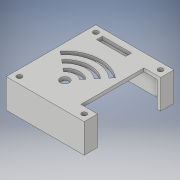
# Autodesk Inventor part: Box1_Top
Saved by Autodesk Inventor 2017 (Build 210142000, 142)
## iProperties
Created: 2017-11-12
Part Number: Box1_Top
Material: Generic
Document SubType Name: Modeling
Designer: Arthur Bondar
Density: 1 g/cm^3
Appearance: Default
Author: Arthur Bondar
Autodesk Inventor part; units mm, degrees
ref_plane "YZ Plane" through (0, 0, 0) normal (1, 0, 0) x (0, 1, 0)
ref_plane "XZ Plane" through (0, 0, 0) normal (0, 1, 0) x (-1, 0, 0)
ref_plane "XY Plane" through (0, 0, 0) normal (0, 0, 1) x (1, 0, 0)
sketch "Sketch1" plane through (0, 0, 0) normal (0, 1, 0) x (-1, 0, 0)
  line L0 (23.5, 27) -> (-23.5, 27)
  line L1 (-23.5, -27) -> (23.5, -27)
  line L2 (23.5, -27) -> (23.5, 27)
  line L3 (21.5, 25) -> (-21.5, 25)
  line L4 (-21.5, -25) -> (21.5, -25)
  line L5 (21.5, -25) -> (21.5, 25)
  line L6 (-21.5, -25) -> (-21.5, -19)
  line L7 (-21.5, -19) -> (-23.5, -19)
  line L8 (-21.5, 25) -> (-21.5, 19)
  line L9 (-21.5, 19) -> (-23.5, 19)
  line L10 (-23.5, 27) -> (-23.5, 19)
  line L11 (-23.5, -19) -> (-23.5, -27)
  line L12 (-21.5, 25) -> (-21.5, 19)
  line L13 (-21.5, -19) -> (-21.5, -25)
  dimension "d2" = 47
  dimension "d3" = 54
  dimension "d4" = 43
  dimension "d5" = 50
  dimension "d6" = 6
  dimension "d7" = 6
  constraints: 28 end point, 8 perpendicular, 6 parallel, 2 horizontal
  measures "d2" distance of L1.end L1.start
  measures "d3" distance of L1.start L0.end
  measures "d4" distance of L4.end L4.start
  measures "d5" distance of L4.start L3.end
  measures "d6" distance of L4.start L6.end
  measures "d7" distance of L3.end L8.end
extrude "Extrusion1" add sketch "Sketch1" along normal blind 4.5
sketch "Sketch2" plane through (0, 4.5, 0) normal (0, 1, 0) x (1, 0, 0)
  line L0 (23.5, -27) -> (-23.5, -27)
  line L1 (23.5, 27) -> (-23.5, 27) projected
  line L2 (-23.5, -27) -> (-23.5, 27)
  line L3 (-23.5, 27) -> (23.5, 27)
  line L4 (23.5, 19) -> (23.5, 27) projected
  line L5 (23.5, 27) -> (23.5, 19)
  line L6 (23.5, 19) -> (21.5, 19)
  line L7 (21.5, 25) -> (21.5, 19) projected
  line L8 (21.5, 19) -> (21.5, 25)
  line L9 (21.5, 25) -> (-21.5, 25)
  line L10 (-21.5, -25) -> (-21.5, 25) projected
  line L11 (-21.5, 25) -> (-21.5, -25)
  line L12 (-21.5, -25) -> (21.5, -25)
  line L13 (21.5, -25) -> (21.5, -19)
  line L14 (21.5, -19) -> (23.5, -19)
  line L15 (23.5, -27) -> (23.5, -19) projected
  line L16 (23.5, -19) -> (23.5, -27)
  line L17 (21.5, -25) -> (-21.5, -25) projected
  line L18 (-21.5, -25) -> (-19.5, -25)
  circle A0 centre (-19.5, -23) radius 1.5
  circle A1 centre (-19.5, -23) radius 2
  line L19 (-21.5, 25) -> (-19.5, 25)
  line L20 (-21.5, 25) -> (21.5, 25) projected
  circle A2 centre (-19.5, 23) radius 1.5
  circle A3 centre (-19.5, 23) radius 2
  line L21 (21.5, 25) -> (19.5, 25)
  circle A4 centre (19.5, 23) radius 1.5
  circle A5 centre (19.5, 23) radius 2
  line L22 (21.5, -25) -> (19.5, -25)
  circle A6 centre (19.5, -23) radius 1.5
  circle A7 centre (19.5, -23) radius 2
  point P0 (0, 0)
  dimension "d13" = 2
  constraints: 32 end point, 8 centre point, 7 perpendicular, 5 point on line, 4 coincident, 4 collinear, 4 tangent, 1 horizontal
  measures "d13" distance of L10.end L19.end
extrude "Extrusion2" add sketch "Sketch2" along normal blind 11 contours L0 L2 L1 L4 L6 L7 L9 L10 L12 L13 L14 L15 | A7 | A1 | A5 | A3
sketch "Sketch3" plane through (0, 15.5, 0) normal (0, 1, 0) x (1, 0, 0)
  point P0 (0, 0)
sketch "Sketch4" plane through (0, 15.5, 0) normal (0, 1, 0) x (1, 0, 0)
  circle A0 centre (-19.5, -23) radius 1.5 projected
  circle A1 centre (-19.5, -23) radius 1.5
  circle A2 centre (-19.5, 23) radius 1.5 projected
  circle A3 centre (-19.5, 23) radius 1.5
  arc A4 (19.5, 25) -> (21.5, 23) centre (19.5, 23) ccw projected
  circle A5 centre (19.5, 23) radius 1.5
  circle A6 centre (19.5, -23) radius 1.5 projected
  circle A7 centre (19.5, -23) radius 1.5
  line L0 (23.5, 27) -> (-23.5, 27) projected
  line L1 (23.5, -27) -> (-23.5, -27)
  line L2 (-23.5, -27) -> (-23.5, 27)
  line L3 (-23.5, 27) -> (23.5, 27)
  line L4 (23.5, 19) -> (23.5, 27) projected
  line L5 (23.5, 19) -> (13.5, 19)
  line L6 (23.5, -27) -> (23.5, -19) projected
  line L7 (23.5, -19) -> (13.5, -19)
  line L8 (13.5, -19) -> (13.5, 19)
  line L9 (23.5, 27) -> (23.5, 19)
  line L10 (23.5, -19) -> (23.5, -27)
  line L11 (-23.5, 27) -> (-23.5, -27) projected
  line L12 (-21.5, -25) -> (-21.5, 25) projected
  line L13 (-19.5, 25) -> (19.5, 25) projected
  line L14 (-15.5, 23) -> (2, 23)
  line L15 (2, 23) -> (2, 19.5)
  line L16 (2, 19.5) -> (-15.5, 19.5)
  line L17 (-15.5, 19.5) -> (-15.5, 23)
  point P0 (0, 0)
  dimension "d24" = 10
  dimension "d25" = 10
  dimension "d31" = 17.5
  dimension "d32" = 3.5
  constraints: 24 end point, 5 parallel, 4 centre point, 4 coincident, 4 horizontal, 2 perpendicular
  measures "d24" distance of L4.start L5.end
  measures "d25" distance of L6.end L7.end
  measures "d31" distance of L15.end L16.end
  measures "d32" distance of L14.end L15.end
extrude "Extrusion3" add sketch "Sketch4" along normal blind 2
sketch "Sketch5" plane through (-23.5, 0, -27) normal (-1, 0, 0) x (0, 0, 1)
  point P0 (27, 0)
sketch "Sketch6" plane through (-23.5, 0, -27) normal (-1, 0, 0) x (0, 0, 1)
  point P0 (27, 0)
sketch "Sketch7" plane through (0, 17.5, 0) normal (0, 1, 0) x (1, 0, 0)
  circle A0 centre (-3.8686, -11.2916) radius 2.7
  arc A1 (0.181, -6.4655) -> (-8.6946, -7.242) centre (-3.8686, -11.2916) ccw
  arc A2 (1.9165, -4.3972) -> (-10.763, -5.5065) centre (-3.8686, -11.2916) ccw
  arc A3 (4.2306, -1.6394) -> (-13.5207, -3.1924) centre (-3.8686, -11.2916) ccw
  arc A4 (5.9661, 0.4289) -> (-15.589, -1.4569) centre (-3.8686, -11.2916) ccw
  arc A5 (8.2801, 3.1867) -> (-18.3468, 0.8571) centre (-3.8686, -11.2916) ccw
  arc A6 (10.0162, 5.2557) -> (-20.2878, 2.7444) centre (-3.8686, -11.2916) ccw
  line L0 (-20.2878, 2.7444) -> (-20.4151, 2.5927)
  line L1 (-20.4151, 2.5927) -> (-20.2871, 2.4853)
  line L2 (-18.3468, 0.8571) -> (-20.2871, 2.4853)
  line L3 (-13.5207, -3.1924) -> (-15.589, -1.4569)
  line L4 (-8.6946, -7.242) -> (-10.763, -5.5065)
  line L5 (0.181, -6.4655) -> (1.9165, -4.3972)
  line L6 (4.2306, -1.6394) -> (5.9661, 0.4289)
  line L7 (8.2801, 3.1867) -> (10.0162, 5.2557)
  dimension "d58" = 5.4
  constraints: 16 end point, 12 point on circle, 7 centre point, 6 coincident, 1 perpendicular
  measures "d58" diameter of A0
extrude "Extrusion4" cut sketch "Sketch7" against normal through all
body "Solid1"
